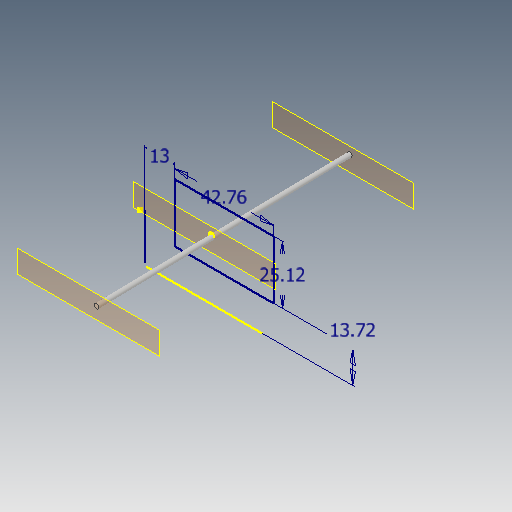
# Autodesk Inventor part: 00_Anybeam_Nebra_HAT_RAY
Saved by Autodesk Inventor 2019.4 (Build 234330000, 330)
## iProperties
Created: 2020-10-22
Part Number: 00_Anybeam_Nebra_HAT_RAY
Material: Generic
Document SubType Name: Modeling
Designer: diederichbenedict
Density: 1 g/cm^3
Appearance: Default
Author: diederichbenedict
Autodesk Inventor part; units mm, degrees
ref_plane "YZ Plane" through (0, 0, 0) normal (1, 0, 0) x (0, 1, 0)
ref_plane "XZ Plane" through (0, 0, 0) normal (0, 1, 0) x (-1, 0, 0)
ref_plane "XY Plane" through (0, 0, 0) normal (0, 0, 1) x (1, 0, 0)
ref_plane "Work Plane1" through (0, 0, -10) normal (0, 0, 1) x (1, 0, 0)
sketch "Sketch1" plane through (0, 0, -10) normal (0, 0, 1) x (1, 0, 0)
  circle A0 centre (30.8569, 6.2439) radius 1 projected
  line L0 (29.2243, 4.7917) -> (32.4895, 4.7917)
  line L1 (32.4895, 4.7917) -> (32.4895, 7.6961)
  line L2 (32.4895, 7.6961) -> (29.2243, 7.6961)
  line L3 (29.2243, 7.6961) -> (29.2243, 4.7917)
  line L4 (29.2243, 4.7917) -> (32.4895, 7.6961) construction
  line L5 (32.4895, 4.7917) -> (29.2243, 7.6961) construction
  point P0 (0, 0)
  constraints: 12 end point, 2 midpoint, 2 parallel, 1 horizontal, 1 perpendicular
ref_plane "Work Plane2" through (0, 0, 50) normal (0, 0, 1) x (1, 0, 0)
sketch "Sketch2" plane through (0, 0, 50) normal (0, 0, 1) x (1, 0, 0)
  circle A0 centre (30.8569, 6.2439) radius 1 projected
  line L0 (15, -5.9361) -> (57.76, -5.9361)
  line L1 (57.76, -5.9361) -> (57.76, 19.1839)
  line L2 (57.76, 19.1839) -> (15, 19.1839)
  line L3 (15, 19.1839) -> (15, -5.9361)
  line L4 (2.8569, -19.6561) -> (52.8569, -19.6561) projected
  line L5 (2, -18.27) -> (2, 1)
  point P0 (0, 0)
  dimension "d0" = 42.76
  dimension "d1" = 25.12
  dimension "d2" = 13
  dimension "d3" = 13.72
  constraints: 10 end point, 2 parallel, 1 horizontal, 1 perpendicular, 1 vertical, 2 other
  measures "d0" distance of L2.end L1.end
  measures "d1" distance of L1.end L0.end
  measures "d2" distance between parallel lines of L3 L5
  measures "d3" distance between parallel lines of L4 L0
ref_plane "Work Plane3" through (0, 0, 100) normal (0, 0, 1) x (1, 0, 0)
sketch "Sketch3" plane through (0, 0, 100) normal (0, 0, 1) x (1, 0, 0)
  line L0 (-31.32, 39.1939) -> (94.02, 39.1939)
  line L1 (94.02, 39.1939) -> (94.02, -29.8061)
  line L2 (94.02, -29.8061) -> (-31.32, -29.8061)
  line L3 (-31.32, -29.8061) -> (-31.32, 39.1939)
  line L4 (2.8569, -19.6561) -> (52.8569, -19.6561) projected
  line L5 (2, -18.27) -> (2, 1) projected
  line L6 (-31.32, 39.1939) -> (94.02, -29.8061) construction
  line L7 (94.02, 39.1939) -> (-31.32, -29.8061) construction
  circle A0 centre (31.35, 4.6939) radius 1
  point P0 (0, 0)
  dimension "d4" = 125.34
  dimension "d5" = 69
  dimension "d6" = 10.15
  dimension "d7" = 33.32
  dimension "d8" = 2
  constraints: 12 end point, 2 parallel, 1 centre point, 1 horizontal, 1 midpoint, 1 perpendicular
  measures "d4" distance of L1.end L2.end
  measures "d5" distance of L0.end L1.end
  measures "d6" distance between parallel lines of L4 L2
  measures "d7" distance between parallel lines of L5 L3
  measures "d8" diameter of A0
loft "Loft1" add profiles "Sketch1", "Sketch3" contours A0 / A0
body "Solid1"
